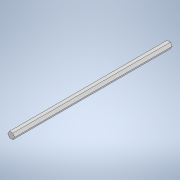
# Autodesk Inventor part: PX9200-25
Saved by Autodesk Inventor 2022.3 (Build 263350000, 350)
## iProperties
Created: 2022-07-21
Part Number: PX9200-25
Material: Generic
Document SubType Name: Modeling
Designer: luis_
Density: 1 g/cm^3
Appearance: Default
Author: luis_
Autodesk Inventor part; units mm, degrees
ref_plane "YZ Plane" through (0, 0, 0) normal (1, 0, 0) x (0, 1, 0)
ref_plane "XZ Plane" through (0, 0, 0) normal (0, 1, 0) x (-1, 0, 0)
ref_plane "XY Plane" through (0, 0, 0) normal (0, 0, 1) x (1, 0, 0)
sketch "Sketch1" plane through (0, 0, 0) normal (0, 0, 1) x (1, 0, 0)
  line L0 (4.6188, 0) -> (2.3094, -4)
  line L1 (2.3094, -4) -> (-2.3094, -4)
  line L2 (-2.3094, -4) -> (-4.6188, 0)
  line L3 (-4.6188, 0) -> (-2.3094, 4)
  line L4 (-2.3094, 4) -> (2.3094, 4)
  line L5 (2.3094, 4) -> (4.6188, 0)
  point P0 (0, 0)
  point P1 (0, 0)
  point P2 (0, 4)
  dimension "d0" = 4
  constraints: 12 end point, 1 coincident, 1 midpoint, 13 other
  measures "d0" distance of point (0, 4) point (0, 0)
extrude "Extrusion1" add sketch "Sketch1" along normal blind 220
body "Solid1"
